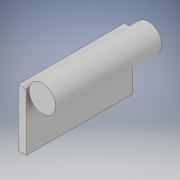
# Autodesk Inventor part: kes
Saved by Autodesk Inventor 2019 (Build 230136000, 136)
## iProperties
Created: 2020-04-03
Part Number: kes
Material: Generic
Document SubType Name: Modeling
Designer: laca
Density: 1 g/cm^3
Appearance: Default
Author: laca
Autodesk Inventor part; units mm, degrees
ref_plane "YZ Plane" through (0, 0, 0) normal (1, 0, 0) x (0, 1, 0)
ref_plane "XZ Plane" through (0, 0, 0) normal (0, 1, 0) x (-1, 0, 0)
ref_plane "XY Plane" through (0, 0, 0) normal (0, 0, 1) x (1, 0, 0)
sketch "Sketch1" plane through (0, 0, 0) normal (0, 0, 1) x (1, 0, 0)
  circle A0 centre (0, 0) radius 25
  line L0 (0, 0) -> (-45.5599, 0)
  line L1 (-45.5599, 0) -> (-45.5599, -94.5606)
  line L2 (-45.5599, 0) -> (0, 0)
  line L3 (-45.5599, 0) -> (-30, 0)
  line L4 (-30, 0) -> (-30, -107.9074)
  line L5 (-30, -107.9074) -> (-45.5599, -107.9074)
  line L6 (-45.5599, -107.9074) -> (-45.5599, 0)
  line L7 (-30, -107.9074) -> (0, 0)
  dimension "d0" = 50
  dimension "d7" = 112
  dimension "d8" = 30
  constraints: 16 end point, 3 horizontal, 2 parallel, 1 centre point, 1 coincident, 1 perpendicular, 1 vertical
  measures "d0" diameter of A0
  measures "d7" distance of L4.end L0.start
  measures "d8" distance from line of point (0, 0) L4
extrude "Extrusion1" add sketch "Sketch1" along normal blind 200 contours A0 L7 L0 | L0 L7 A0 | L4 L5 L6 L1 L0
body "Solid1"
